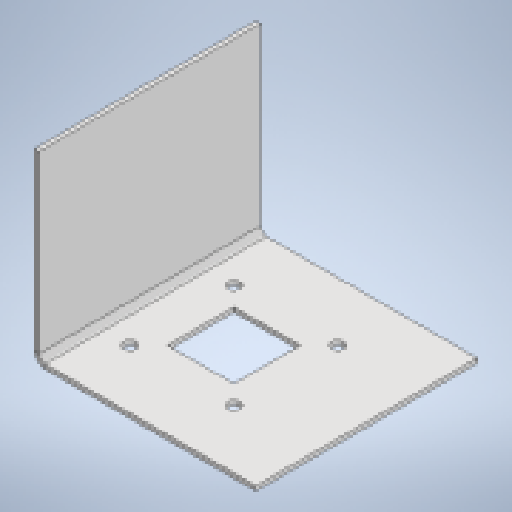
# Autodesk Inventor part: PNS 753 FDS 1200 FLANGE 2 up
Saved by Autodesk Inventor 2025 (Build 290162010, 162A)
## iProperties
Created: 2025-06-24
Part Number: PNS 753 FDS 1200 FLANGE 2 up
Material: Stainless Steel
Description: DIE16(5)|\ 90°|corrY -___°|X_____|bom___
Document SubType Name: Sheet Metal
Designer: pokla
Mass: 971.211 g
Surface Area: 1239.79 cm^2
Volume: 121.401 cm^3
Density: 8 g/cm^3
Flat Pattern Width: 18.0202 cm
Flat Pattern Length: 10 cm
Flat Pattern Area: 180.202 cm^2
Sheet Metal Rule: AISI304 2mm Die16
Sheet Metal Width: 180,202 mm
Sheet Metal Length: 100,000 mm
Sheet Metal Area: 18020,199 mm^2
Appearance: Default
d177: 30,000 mm
d178: 30,000 mm
Author: user
Autodesk Inventor part; units mm, degrees
ref_plane "YZ Plane" through (0, 0, 0) normal (1, 0, 0) x (0, 1, 0)
ref_plane "XZ Plane" through (0, 0, 0) normal (0, 1, 0) x (-1, 0, 0)
ref_plane "XY Plane" through (0, 0, 0) normal (0, 0, 1) x (1, 0, 0)
sketch "Sketch1" plane through (0, 0, 0) normal (0, 0, 1) x (1, 0, 0)
  line L0 (-50, -50) -> (50, -50)
  line L1 (50, -50) -> (50, 50)
  line L2 (50, 50) -> (-50, 50)
  line L3 (-50, 50) -> (-50, -50)
  line L4 (-50, -50) -> (50, 50) construction
  line L5 (50, -50) -> (-50, 50) construction
  point P0 (0, 0)
  dimension "d154" = 100
  dimension "d155" = 100
  measures "d154" distance of L1.end L2.end
  measures "d155" distance of L0.end L1.end
extrude "Plate5" add sketch "Sketch1" along normal blind 2
sketch "Sketch9" plane through (0, 0, 0) normal (0, 0, -1) x (-1, 0, 0)
  line L0 (25, -15) -> (-5, -15)
  line L1 (-5, -15) -> (-5, 15)
  line L2 (-5, 15) -> (25, 15)
  line L3 (25, 15) -> (25, -15)
  line L4 (25, -15) -> (-5, 15) construction
  line L5 (-5, -15) -> (25, 15) construction
  circle A0 centre (33.4853, -23.4853) radius 2.75
  circle A1 centre (-13.4853, -23.4853) radius 2.75
  circle A2 centre (-13.4853, 23.4853) radius 2.75
  circle A3 centre (33.4853, 23.4853) radius 2.75
  circle A4 centre (10, 0) radius 33.2132 construction
  line L6 (-5, -15) -> (-13.4853, -23.4853) construction
  line L7 (50, 50) -> (50, -50) projected
  line L8 (-50, -50) -> (-50, 50) projected
  line L9 (50, -50) -> (-50, -50) projected
  line L10 (50, 50) -> (50, -50) projected
  line L11 (-50, 50) -> (50, 50) projected
  point P0 (0, 0)
  dimension "d173" = 30
  dimension "d174" = 30
  dimension "d175" = 5.5
  dimension "d176" = 12
  dimension "d179" = 40
  dimension "d180" = 50
  constraints: 14 end point, 5 centre point, 4 point on circle, 4 point on line, 3 equal radius, 2 midpoint, 2 parallel, 1 coincident, 1 horizontal, 1 perpendicular
  measures "d173" distance of L0.start L6.start
  measures "d174" distance of L6.start L1.end
  measures "d175" diameter of A0
  measures "d176" distance of L6.end L6.start
  measures "d179" distance from line of point (10, 0) L7
  measures "d180" distance from line of L11 point (10, 0)
sketch "Sketch7" plane through (-48, -50, 0) normal (-1, 0, 0) x (0, -1, 0)
  line L0 (-100, 0) -> (0, 0)
  line L1 (0, 0) -> (0, 84)
  line L2 (0, 84) -> (-100, 84)
  line L3 (-100, 84) -> (-100, 0)
  constraints: 6 end point, 1 horizontal, 1 perpendicular, 1 vertical
edge flange "Flange3" height 84 angle 90 thickness 2 bend radius 2.75 thickness toward (-1, 0, 0) relief round relief width 2 relief depth 1 edges at (-50, 0, 2) wall of the first edge with corners at (-48, 50, 0) (-48, -50, 0) (-48, -50, 84) (-48, 50, 84)
bend "Bend3"
corner "Corner3"
extrude "Extrusion3" cut sketch "Sketch9" against normal blind 10 contours L0 L1 L2 L3 | A0 | A1 | A2 | A3
body "Solid3"
